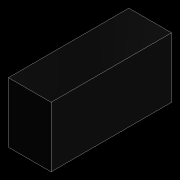
# Autodesk Inventor part: 300 mAh 4s Mockup Battery
Saved by Autodesk Inventor 2022 (Build 260153000, 153)
## iProperties
Created: 2022-08-01
Part Number: 300 mAh 4s Mockup Battery
Material: Generic
Document SubType Name: Modeling
Designer: tandu
Density: 1.73611 g/cm^3
Appearance: Aluminum - Polished(1)
Mass: 34 g
Surface Area: 47.52 cm^2
Volume: 19.584 cm^3
Author: tandu
Autodesk Inventor part; units mm, degrees
ref_plane "YZ Plane" through (0, 0, 0) normal (1, 0, 0) x (0, 1, 0)
ref_plane "XZ Plane" through (0, 0, 0) normal (0, 1, 0) x (-1, 0, 0)
ref_plane "XY Plane" through (0, 0, 0) normal (0, 0, 1) x (1, 0, 0)
sketch "Sketch1" plane through (0, 0, 0) normal (0, 1, 0) x (-1, 0, 0)
  line L0 (-8.5, 24) -> (8.5, 24)
  line L1 (8.5, 24) -> (8.5, -24)
  line L2 (8.5, -24) -> (-8.5, -24)
  line L3 (-8.5, -24) -> (-8.5, 24)
  line L4 (-8.5, 24) -> (8.5, -24) construction
  line L5 (8.5, 24) -> (-8.5, -24) construction
  point P0 (0, 0)
  dimension "d0" = 17
  dimension "d1" = 48
  constraints: 12 end point, 2 midpoint, 2 parallel, 1 horizontal, 1 perpendicular
  measures "d0" distance of L1.end L2.end
  measures "d1" distance of L0.end L1.end
extrude "Extrusion1" add sketch "Sketch1" along normal mid plane 24
body "Solid1"
